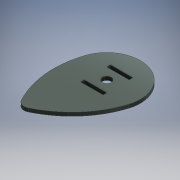
# Autodesk Inventor part: leva00
Saved by Autodesk Inventor 2016 (Build 200138000, 138)
## iProperties
Created: 2016-09-20
Part Number: leva00
Material: Madera (abedul)
Document SubType Name: Modeling
Designer: i95sa
Density: 0.55 g/cm^3
Appearance: Gris plomo - Pulido
Author: i95sa
Autodesk Inventor part; units mm, degrees
ref_plane "YZ Plane" through (0, 0, 0) normal (1, 0, 0) x (0, 1, 0)
ref_plane "XZ Plane" through (0, 0, 0) normal (0, 1, 0) x (-1, 0, 0)
ref_plane "XY Plane" through (0, 0, 0) normal (0, 0, 1) x (1, 0, 0)
sketch "Boceto1" plane through (0, 0, 0) normal (0, 0, 1) x (1, 0, 0)
  arc A0 (11.6499, 35.8548) -> (-11.6499, -35.8548) centre (0, 0) ccw
  arc A1 (-17.9283, -55.1778) -> (-23.3052, -71.7261) centre (-20.6168, -63.452) ccw
  line L0 (-24.0836, -74.1217) -> (-32.3578, -71.4333)
  line L1 (-35.7143, 12.0739) -> (-49.5046, 16.5546)
  line L2 (-49.5046, 16.5546) -> (-32.3578, -71.4333)
  line L3 (-32.3578, -71.4333) -> (-39.0143, -37.2758)
  arc A2 (-35.7143, 12.0739) -> (-39.0143, -37.2758) centre (55.6772, -18.8226) ccw
  arc A3 (-39.0143, -37.2758) -> (-28.3005, -67.5324) centre (67.9138, -16.438) ccw
  line L4 (0.8961, 2.7581) -> (11.6499, 35.8548)
  line L5 (-0.8961, -2.7581) -> (-24.0836, -74.1217)
  arc A4 (-11.6499, -35.8548) -> (11.6499, 35.8548) centre (0, 0) ccw
  arc A5 (-23.3052, -71.7261) -> (-17.9283, -55.1778) centre (-20.6168, -63.452) ccw
  line L6 (-24.0836, -74.1217) -> (-15.8094, -76.8102)
  line L7 (35.9903, -11.2244) -> (49.7806, -15.7051)
  line L8 (49.7806, -15.7051) -> (-15.8094, -76.8102)
  line L9 (-15.8094, -76.8102) -> (9.653, -53.0888)
  arc A6 (9.653, -53.0888) -> (35.9903, -11.2244) centre (-56.1074, 17.4984) ccw
  arc A7 (-16.7989, -71.2695) -> (9.653, -53.0888) centre (-64.6054, 26.6201) ccw
  dimension "d0" = 75.4
  dimension "d6" = 17.4
  dimension "d7" = 8.7
  dimension "d8" = 14.5
  dimension "d9" = 34.8
  constraints: 20 end point, 20 point on circle, 8 centre point, 6 symmetric about line, 5 point on line, 4 tangent, 1 collinear, 4 other
  measures "d0" diameter of A0
  measures "d6" diameter of A1
  measures "d7" distance of L0.start L0.end
  measures "d8" distance of L1.start L1.end
  measures "d9" distance of L0.end L3.end
extrude "Extrusión2" add sketch "Boceto1" along normal blind 4 contours A4 A0 | A0 L5 A1 A3 A2 | A6 A7 A5 L5 A4 | L5 A1 | A5 L5
sketch "Boceto2" plane through (0, 0, 4) normal (0, 0, 1) x (1, 0, 0)
  line L0 (0, 0) -> (0, 12.5)
  line L1 (0, 12.5) -> (-12.5, 12.5)
  line L2 (-12.5, 12.5) -> (-12.5, 16.7)
  line L3 (-12.5, 16.7) -> (12.5, 16.7)
  line L4 (12.5, 16.7) -> (12.5, 12.5)
  line L5 (12.5, 12.5) -> (0, 12.5)
  line L6 (0, 0) -> (12.5, 0)
  line L7 (0, 0) -> (0, -12.5)
  line L8 (0, -12.5) -> (-12.5, -12.5)
  line L9 (-12.5, -12.5) -> (-12.5, -16.7)
  line L10 (-12.5, -16.7) -> (12.5, -16.7)
  line L11 (12.5, -16.7) -> (12.5, -12.5)
  line L12 (12.5, -12.5) -> (0, -12.5)
  circle A0 centre (0, 0) radius 5
  dimension "d24" = 12.5
  dimension "d25" = 12.5
  dimension "d26" = 4.2
  dimension "d27" = 25
  dimension "d28" = 10
  constraints: 26 end point, 5 perpendicular, 5 symmetric about line, 3 point on line, 1 centre point, 1 coincident, 1 parallel, 1 vertical
  measures "d24" distance of L0.start L0.end
  measures "d25" distance of L0.end L1.end
  measures "d26" distance of L1.end L2.end
  measures "d27" distance of L2.end L3.end
  measures "d28" diameter of A0
extrude "Extrusión3" cut sketch "Boceto2" against normal blind 4
